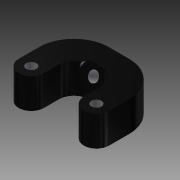
# Autodesk Inventor part: Mount
Saved by Autodesk Inventor 2015 (Build 190159000, 159)
## iProperties
Created: 2017-01-08
Part Number: Mount
Material: Generic
Document SubType Name: Modeling
Designer: Ernest
Density: 1 g/cm^3
Appearance: Default
Author: Ernest
Autodesk Inventor part; units mm, degrees
ref_plane "YZ Plane" through (0, 0, 0) normal (1, 0, 0) x (0, 1, 0)
ref_plane "XZ Plane" through (0, 0, 0) normal (0, 1, 0) x (-1, 0, 0)
sketch "Sketch1" plane through (0, 0, 0) normal (0, 0, 1) x (1, 0, 0)
  circle A0 centre (0, 0) radius 5
  circle A1 centre (65, 0) radius 5
  circle A2 centre (0, 0) radius 12.5
  circle A3 centre (65, 0) radius 12.5
  line L0 (22.5, 9.5) -> (42.5, 9.5)
  line L1 (42.5, 9.5) -> (42.5, -10.5)
  line L2 (42.5, -10.5) -> (22.5, -10.5)
  line L3 (22.5, -10.5) -> (22.5, 9.5)
  line L4 (0, 0) -> (65, 0) construction
  line L5 (32.5, 0) -> (32.5, 30) construction
  line L6 (27.5, 30) -> (37.5, 30)
  line L7 (12.5, 0) -> (12.5, 15)
  line L8 (52.5, 0) -> (52.5, 15)
  arc A4 (27.5, 30) -> (12.5, 15) centre (27.5, 15) ccw
  arc A5 (52.5, 15) -> (37.5, 30) centre (37.5, 15) ccw
  line L9 (-12.5, 0) -> (-12.5, 20)
  line L10 (77.5, 0) -> (77.5, 20)
  line L11 (22.5, 55) -> (42.5, 55)
  arc A6 (22.5, 55) -> (-12.5, 20) centre (22.5, 20) ccw
  arc A7 (77.5, 20) -> (42.5, 55) centre (42.5, 20) ccw
  point P0 (22.5, 30)
  point P1 (42.5, 30)
  dimension "d0" = 10
  dimension "d1" = 10
  dimension "d2" = 65
  dimension "d3" = 25
  dimension "d4" = 25
  dimension "d5" = 22.5
  dimension "d6" = 22.5
  dimension "d7" = 9.5
  dimension "d8" = 10.5
  dimension "d11" = 20
  dimension "d12" = 10
  dimension "d13" = 30
  dimension "d14" = 15
  dimension "d15" = 55
  dimension "d16" = 35
  constraints: 24 end point, 12 point on circle, 12 tangent, 8 centre point, 4 horizontal, 4 point on line, 3 coincident, 3 perpendicular, 3 vertical, 2 equal radius, 2 midpoint, 2 parallel
  measures "d0" diameter of A0
  measures "d1" diameter of A1
  measures "d2" distance of A1.centre point (0, 0)
  measures "d3" diameter of A2
  measures "d4" diameter of A3
  measures "d5" distance from line of L3 point (0, 0)
  measures "d6" distance from line of L1 A1.centre
  measures "d7" distance from line of L0 point (0, 0)
  measures "d8" distance from line of point (0, 0) L2
  measures "d11" distance of point (22.5, 30) point (42.5, 30)
  measures "d12" distance of L5.end point (22.5, 30)
  measures "d13" distance of L5.start L5.end
  measures "d14" radius of A4
  measures "d15" distance from line of L11 L5.start
  measures "d16" radius of A6
extrude "Extrusion1" add sketch "Sketch1" along normal blind 30 contours A2 | A2 L9 A6 L11 A7 L10 A3 L8 A5 L6 A4 L7 | A3
ref_plane "Work Plane1" through (42.5, 55, 0) normal (0, 0.8660254, -0.5) x (-1, 0, 0)
sketch "Sketch2" plane through (42.5, 55, 0) normal (0, 0.8660254, -0.5) x (-1, 0, 0)
  line L0 (0, 0) -> (20, 0) projected
  line L1 (20, 0) -> (20, 25.9808) projected
  line L2 (0, 25.9808) -> (20, 25.9808) projected
  line L3 (0, 0) -> (0, 25.9808) projected
  line L4 (15, -12.5) -> (5, -12.5) projected
  line L5 (5, -12.5) -> (5, 13.4808) projected
  line L6 (15, 13.4808) -> (5, 13.4808) projected
  line L7 (15, -12.5) -> (15, 13.4808) projected
  circle A0 centre (10, 6.7404) radius 5
  circle A1 centre (10, 6.7404) radius 12.5
  point P0 (42.5, -27.5)
  dimension "d20" = 38.4808
  dimension "d21" = 19.2404
  dimension "d22" = 20
  dimension "d23" = 10
  dimension "d24" = 10
  dimension "d25" = 25
  constraints: 2 centre point, 1 coincident
  measures "d20" distance between parallel lines of L4 L2
  measures "d21" distance from line of L2 A0.centre
  measures "d22" distance of L2.start L1.end
  measures "d23" distance from line of L1 A0.centre
  measures "d24" diameter of A0
  measures "d25" diameter of A1
extrude "Extrusion6" cut sketch "Sketch2" against normal blind 55.75 contours A0
extrude "Extrusion7" add sketch "Sketch2" against normal blind 39.25 contours L3 A1 L1 L0 L7 L6 L5 | L0 L5 A1 L3 | L5 A0 L7 L0 | L0 L7 A1 L5 | L0 L1 A1 L7 | L5 L6 L7 A0
sketch "Sketch5" plane through (32.5, 24.3787, 25.4623) normal (0, -0.8660254, 0.5) x (-1, 0, 0)
  circle A0 centre (0, 0) radius 5 projected
  circle A1 centre (0, 0) radius 12.5 projected
  point P0 (32.5, 34.2404)
extrude "Extrusion8" cut sketch "Sketch5" against normal blind 6
sketch "Sketch6" plane through (22.5, 55, 30) normal (0, 1, 0) x (1, 0, 0)
  ellipse E0 centre (10, 7.5377) end of major axis (22.5, 7.5377) minor radius 10.8253 (1.0281, 0) -> (18.9719, 0) ccw projected
  line L0 (1.0281, 0) -> (18.9719, 0) projected
  point P0 (-22.5, 30)
  constraints: 1 other
extrude "Extrusion9" cut sketch "Sketch6" against normal blind 41
fillet "Fillet3" radius 1.5 2 edges at (20.4586, 31.2539, 25.3665) (44.5414, 31.2539, 25.3665)
equation "\"d12\" = 0.5 * d11"
equation "\"d15\" = d13 + d3"
equation "\"d21\" = 0.5 * d20"
equation "\"d23\" = 0.5 * d22"
body "Solid1"
